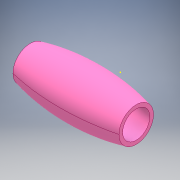
# Autodesk Inventor part: roller rubber test
Saved by Autodesk Inventor 2018 (Build 220112000, 112)
## iProperties
Created: 2017-09-19
Part Number: roller rubber test
Material: Generic
Document SubType Name: Modeling
Designer: M227958
Density: 1 g/cm^3
Appearance: Pink
Author: M227958
Autodesk Inventor part; units mm, degrees
note: some values were not read from the file. Chosen so that the rebuilt part matches the saved one: offset side.
ref_plane "YZ Plane" through (0, 0, 0) normal (1, 0, 0) x (0, 1, 0)
ref_plane "XZ Plane" through (0, 0, 0) normal (0, 1, 0) x (-1, 0, 0)
ref_plane "Work Plane1" through (0, 0, 0) normal (0, -0.8660254, 0.5) x (1, 0, 0)
sketch "Sketch1" plane through (0, 0, 0) normal (0, -0.8660254, 0.5) x (1, 0, 0)
  circle A0 centre (0, 0) radius 97 construction
  dimension "d1" = 194
  constraints: 1 centre point, 1 coincident
  measures "d1" diameter of A0
sketch "Sketch2" plane through (0, 0, 0) normal (0, 1, 0) x (-1, 0, 0)
  point P0 (0, 0)
sketch "Sketch3" plane through (0, 0, 0) normal (0, 0, 1) x (1, 0, 0)
  ellipse E0 centre (0, 0) end of major axis (97, 0) minor radius 48.5 construction
  circle A0 centre (0, -31.5) radius 17
  line L0 (0, -31.5) -> (44.8665, -31.5)
  line L1 (0, -43) -> (44.8665, -43) construction
  line L2 (0, -31.5) -> (-44.8665, -31.5)
  line L3 (0, -43) -> (-44.8665, -43) construction
  line L4 (44.8665, -43) -> (44.8665, -31.5)
  line L5 (-44.8665, -43) -> (-44.8665, -31.5)
  arc A1 (-44.8665, -43) -> (44.8665, -43) centre (0, 137.25) ccw
  line L6 (-44.8665, -43) -> (-44.8665, -46.0983)
  line L7 (44.8665, -43) -> (44.8665, -46.0983)
  spline S0 degree 5 poles (100, 0) (99.9999, 3.1962) (99.5318, 6.3955) (98.5918, 9.4943) (95.7738, 15.7772) (91.5666, 21.2452) (89.0457, 23.9075) (83.085, 29.252) (76.3752, 33.6319) (72.5885, 35.7652) (64.204, 39.8925) (55.4318, 43.1228) (50.6609, 44.6282) (40.5654, 47.3501) (30.2808, 49.2437) (24.8806, 50.0245) (13.8731, 51.2082) (2.8088, 51.5996) (-2.8083, 51.5996) (-13.8729, 51.2082) (-24.8806, 50.0245) (-30.2811, 49.2437) (-40.5657, 47.3501) (-50.6612, 44.6281) (-55.432, 43.1228) (-64.2039, 39.8925) (-72.5882, 35.7654) (-76.3748, 33.632) (-83.0849, 29.2523) (-89.0457, 23.9073) (-91.5669, 21.2454) (-95.774, 15.7761) (-98.5921, 9.4944) (-99.5318, 6.3937) (-100.4682, 0) (-99.5318, -6.3937) (-98.5921, -9.4944) (-95.774, -15.7761) (-91.5669, -21.2454) (-89.0457, -23.9073) (-83.0849, -29.2523) (-76.3748, -33.632) (-72.5882, -35.7654) (-64.2039, -39.8925) (-55.432, -43.1228) (-50.6612, -44.6281) (-40.5657, -47.3501) (-30.2811, -49.2437) (-24.8806, -50.0245) (-13.8729, -51.2082) (-2.8083, -51.5996) (2.8088, -51.5996) (13.8731, -51.2082) (24.8806, -50.0245) (30.2808, -49.2437) (40.5654, -47.3501) (50.6609, -44.6282) (55.4318, -43.1228) (64.204, -39.8925) (72.5885, -35.7652) (76.3752, -33.6319) (83.085, -29.252) (89.0457, -23.9075) (91.5666, -21.2452) (95.7738, -15.7772) (98.5918, -9.4943) (99.5318, -6.3955) (99.9999, -3.1962) (100, 0) knots 0 0 0 0 0 0 0.032702 0.032702 0.032702 0.070029 0.070029 0.070029 0.114401 0.114401 0.114401 0.165518 0.165518 0.165518 0.22129 0.22129 0.22129 0.278709 0.278709 0.278709 0.334483 0.334483 0.334483 0.385599 0.385599 0.385599 0.42997 0.42997 0.42997 0.4673 0.4673 0.4673 0.5 0.5 0.5 0.5327 0.5327 0.5327 0.57003 0.57003 0.57003 0.614401 0.614401 0.614401 0.665517 0.665517 0.665517 0.721291 0.721291 0.721291 0.77871 0.77871 0.77871 0.834482 0.834482 0.834482 0.885599 0.885599 0.885599 0.929971 0.929971 0.929971 0.967298 0.967298 0.967298 1 1 1 1 1 1
  dimension "d13" = 3
  dimension "d3" = 11.5
  constraints: 16 end point, 4 horizontal, 2 centre point, 2 perpendicular, 2 point on circle, 2 vertical, 1 horizontal alignment, 6 other
  measures "d3" distance of L0.start L1.start
revolve "Revolution1" [suppressed]
sketch "Sketch4" plane through (-44.8665, -31.5, 0) normal (-1, 0, 0) x (0, 0, 1)
  circle A0 centre (0, 0) radius 9.5
  point P0 (0, 31.5)
  dimension "d5" = 19
  constraints: 1 centre point
  measures "d5" diameter of A0
extrude "Extrusion1" [suppressed]
sketch "Sketch5" plane through (-38.8665, -31.5, 0) normal (-1, 0, 0) x (0, 0, 1)
  circle A0 centre (0, 0) radius 4
  point P0 (0, 31.5)
  dimension "d8" = 8
  constraints: 1 centre point
  measures "d8" diameter of A0
extrude "Extrusion2" [suppressed]
sketch "Sketch6" plane through (44.8665, -31.5, 0) normal (1, 0, 0) x (0, 0, -1)
  circle A0 centre (0, 0) radius 4 projected
  circle A1 centre (0, 0) radius 9.5
  point P0 (0, 31.5)
  constraints: 1 centre point, 1 coincident
extrude "Extrusion3" [suppressed]
revolve "Revolution2" add sketch "Sketch3" angle 360 about axis through (0, -31.5, 0) along (-1, 0, 0) contours A1 L7 S0 L6
body "Solid1"
